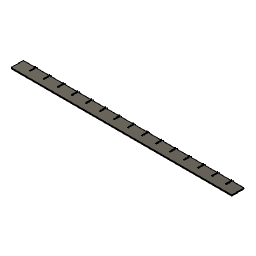
Matrix_Y (Autodesk Fusion 360 design; units mm, degrees)
Autodesk Fusion 360 part; units mm, degrees
other "Base Mesh Feature1"
sketch "Sketch1" plane through (0, 0, 0) normal (0, 0, 1) x (1, 0, 0)
  line L0 (0, 0) -> (252, 0)
  line L1 (252, 0) -> (252, 14)
  line L2 (0, 14) -> (0, 0)
  line L3 (14.5, 15) -> (14.5, 7.35)
  line L4 (14.5, 7.35) -> (13.5, 7.35)
  line L5 (13.5, 7.35) -> (13.5, 15)
  line L6 (13.5, 15) -> (12.5, 15)
  line L7 (30.5, 15) -> (30.5, 7.35)
  line L8 (30.5, 7.35) -> (29.5, 7.35)
  line L9 (29.5, 7.35) -> (29.5, 15)
  line L10 (46.5, 15) -> (46.5, 7.35)
  line L11 (46.5, 7.35) -> (45.35, 7.35)
  line L12 (45.35, 7.35) -> (45.35, 15)
  line L13 (62.5, 15) -> (62.5, 7.35)
  line L14 (62.5, 7.35) -> (61.35, 7.35)
  line L15 (61.35, 7.35) -> (61.35, 15)
  line L16 (78.5, 15) -> (78.5, 7.35)
  line L17 (78.5, 7.35) -> (77.35, 7.35)
  line L18 (77.35, 7.35) -> (77.35, 15)
  line L19 (94.5, 15) -> (94.5, 7.35)
  line L20 (94.5, 7.35) -> (93.35, 7.35)
  line L21 (93.35, 7.35) -> (93.35, 15)
  line L22 (110.5, 15) -> (110.5, 7.35)
  line L23 (110.5, 7.35) -> (109.35, 7.35)
  line L24 (109.35, 7.35) -> (109.35, 15)
  line L25 (126.5, 15) -> (126.5, 7.35)
  line L26 (126.5, 7.35) -> (125.35, 7.35)
  line L27 (125.35, 7.35) -> (125.35, 15)
  line L28 (142.5, 15) -> (142.5, 7.35)
  line L29 (142.5, 7.35) -> (141.35, 7.35)
  line L30 (141.35, 7.35) -> (141.35, 15)
  line L31 (158.5, 15) -> (158.5, 7.35)
  line L32 (158.5, 7.35) -> (157.35, 7.35)
  line L33 (157.35, 7.35) -> (157.35, 15)
  line L34 (174.5, 15) -> (174.5, 7.35)
  line L35 (174.5, 7.35) -> (173.35, 7.35)
  line L36 (173.35, 7.35) -> (173.35, 15)
  line L37 (190.5, 15) -> (190.5, 7.35)
  line L38 (190.5, 7.35) -> (189.35, 7.35)
  line L39 (189.35, 7.35) -> (189.35, 15)
  line L40 (206.5, 15) -> (206.5, 7.35)
  line L41 (206.5, 7.35) -> (205.35, 7.35)
  line L42 (205.35, 7.35) -> (205.35, 15)
  line L43 (222.5, 15) -> (222.5, 7.35)
  line L44 (222.5, 7.35) -> (221.35, 7.35)
  line L45 (221.35, 7.35) -> (221.35, 15)
  line L46 (238.5, 15) -> (238.5, 7.35)
  line L47 (238.5, 7.35) -> (237.35, 7.35)
  line L48 (237.35, 7.35) -> (237.35, 15)
  line L49 (239.5, 15) -> (238.5, 15)
  line L50 (223.5, 15) -> (223.5, 14)
  line L51 (223.5, 14) -> (236.35, 14)
  line L52 (236.35, 14) -> (236.35, 15)
  line L53 (252, 14) -> (239.5, 14)
  line L54 (239.5, 14) -> (239.5, 15)
  line L55 (220.35, 15) -> (220.35, 14)
  line L56 (220.35, 14) -> (207.5, 14)
  line L57 (207.5, 14) -> (207.5, 15)
  line L58 (237.35, 15) -> (236.35, 15)
  line L59 (223.5, 15) -> (222.5, 15)
  line L60 (221.35, 15) -> (220.35, 15)
  line L61 (207.5, 15) -> (206.5, 15)
  line L62 (204.35, 15) -> (204.35, 14)
  line L63 (204.35, 14) -> (191.5, 14)
  line L64 (191.5, 14) -> (191.5, 15)
  line L65 (205.35, 15) -> (204.35, 15)
  line L66 (191.5, 15) -> (190.5, 15)
  line L67 (188.35, 15) -> (188.35, 14)
  line L68 (188.35, 14) -> (175.5, 14)
  line L69 (175.5, 14) -> (175.5, 15)
  line L70 (189.35, 15) -> (188.35, 15)
  line L71 (175.5, 15) -> (174.5, 15)
  line L72 (172.35, 15) -> (172.35, 14)
  line L73 (172.35, 14) -> (159.5, 14)
  line L74 (159.5, 14) -> (159.5, 15)
  line L75 (173.35, 15) -> (172.35, 15)
  line L76 (159.5, 15) -> (158.5, 15)
  line L77 (156.35, 15) -> (156.35, 14)
  line L78 (156.35, 14) -> (143.5, 14)
  line L79 (143.5, 14) -> (143.5, 15)
  line L80 (157.35, 15) -> (156.35, 15)
  line L81 (143.5, 15) -> (142.5, 15)
  line L82 (140.35, 15) -> (140.35, 14)
  line L83 (140.35, 14) -> (127.5, 14)
  line L84 (127.5, 14) -> (127.5, 15)
  line L85 (141.35, 15) -> (140.35, 15)
  line L86 (127.5, 15) -> (126.5, 15)
  line L87 (124.35, 15) -> (124.35, 14)
  line L88 (124.35, 14) -> (111.5, 14)
  line L89 (111.5, 14) -> (111.5, 15)
  line L90 (125.35, 15) -> (124.35, 15)
  line L91 (111.5, 15) -> (110.5, 15)
  line L92 (108.35, 15) -> (108.35, 14)
  line L93 (108.35, 14) -> (95.5, 14)
  line L94 (95.5, 14) -> (95.5, 15)
  line L95 (109.35, 15) -> (108.35, 15)
  line L96 (95.5, 15) -> (94.5, 15)
  line L97 (92.35, 15) -> (92.35, 14)
  line L98 (92.35, 14) -> (79.5, 14)
  line L99 (79.5, 14) -> (79.5, 15)
  line L100 (93.35, 15) -> (92.35, 15)
  line L101 (79.5, 15) -> (78.5, 15)
  line L102 (76.35, 15) -> (76.35, 14)
  line L103 (76.35, 14) -> (63.5, 14)
  line L104 (63.5, 14) -> (63.5, 15)
  line L105 (77.35, 15) -> (76.35, 15)
  line L106 (63.5, 15) -> (62.5, 15)
  line L107 (60.35, 15) -> (60.35, 14)
  line L108 (60.35, 14) -> (47.5, 14)
  line L109 (47.5, 14) -> (47.5, 15)
  line L110 (61.35, 15) -> (60.35, 15)
  line L111 (47.5, 15) -> (46.5, 15)
  line L112 (44.35, 15) -> (44.35, 14)
  line L113 (44.35, 14) -> (31.5, 14)
  line L114 (31.5, 14) -> (31.5, 15)
  line L115 (45.35, 15) -> (44.35, 15)
  line L116 (31.5, 15) -> (30.5, 15)
  line L117 (28.5, 15) -> (28.5, 14)
  line L118 (28.5, 14) -> (15.5, 14)
  line L119 (15.5, 14) -> (15.5, 15)
  line L120 (29.5, 15) -> (28.5, 15)
  line L121 (15.5, 15) -> (14.5, 15)
  line L122 (0, 14) -> (12.5, 14)
  line L123 (12.5, 14) -> (12.5, 15)
  dimension "d2" = 252
  dimension "d5" = 1
  dimension "d6" = 15
  dimension "d7" = 1
  dimension "d8" = 14.85
  dimension "d9" = 1.15
  dimension "d10" = 14.85
  dimension "d11" = 1.15
  dimension "d12" = 14.85
  dimension "d13" = 1.15
  dimension "d14" = 14.85
  dimension "d15" = 1.15
  dimension "d16" = 14.85
  dimension "d17" = 1.15
  dimension "d18" = 14.85
  dimension "d19" = 1.15
  dimension "d20" = 14.85
  dimension "d21" = 1.15
  dimension "d22" = 14.85
  dimension "d23" = 1.15
  dimension "d24" = 14.85
  dimension "d25" = 1.15
  dimension "d26" = 14.85
  dimension "d27" = 1.15
  dimension "d28" = 14.85
  dimension "d29" = 1.15
  dimension "d30" = 14.85
  dimension "d31" = 1.15
  dimension "d32" = 14.85
  dimension "d33" = 1.15
  dimension "d36" = 7.65
  dimension "d37" = 7.65
  dimension "d38" = 7.65
  dimension "d39" = 7.65
  dimension "d40" = 7.65
  dimension "d41" = 7.65
  dimension "d42" = 7.65
  dimension "d43" = 7.65
  dimension "d44" = 7.65
  dimension "d45" = 7.65
  dimension "d46" = 7.65
  dimension "d47" = 7.65
  dimension "d48" = 7.65
  dimension "d49" = 7.65
  dimension "d50" = 7.65
  dimension "d51" = 1
  dimension "d52" = 1
  dimension "d53" = 1
  dimension "d54" = 1
  dimension "d55" = 1
  dimension "d56" = 1
  dimension "d57" = 1
  dimension "d58" = 1
  dimension "d59" = 1
  dimension "d60" = 1
  dimension "d61" = 1
  dimension "d62" = 1
  dimension "d63" = 1
  dimension "d64" = 1
  dimension "d65" = 1
  dimension "d66" = 1
  dimension "d67" = 1
  dimension "d68" = 1
  dimension "d69" = 1
  dimension "d70" = 1
  dimension "d71" = 1
  dimension "d72" = 1
  dimension "d73" = 1
  dimension "d74" = 1
  dimension "d75" = 1
  dimension "d76" = 1
  dimension "d77" = 1
  dimension "d78" = 1
  dimension "d79" = 1
  dimension "d80" = 1
  dimension "d81" = 1
  dimension "d82" = 1
  dimension "d83" = 1
  dimension "d84" = 1
  dimension "d85" = 1
  dimension "d86" = 1
  dimension "d87" = 1
  dimension "d88" = 1
  dimension "d89" = 1
  dimension "d90" = 1
  dimension "d91" = 1
  dimension "d92" = 1
  dimension "d93" = 1
  dimension "d94" = 1
  dimension "d95" = 12.5
  dimension "d96" = 12.5
  constraint horizontal L0
  constraint vertical L1
  constraint horizontal L49
  constraint vertical L2
  constraint coincident L0.start L2.end
  constraint vertical L3
  constraint horizontal L4
  constraint vertical L5
  constraint coincident L5.end L49
  constraint collinear L6 L49
  constraint vertical L7
  constraint horizontal L8
  constraint vertical L9
  constraint coincident L9.end L49
  constraint vertical L10
  constraint horizontal L11
  constraint vertical L12
  constraint coincident L12.end L49
  constraint vertical L13
  constraint horizontal L14
  constraint vertical L15
  constraint coincident L15.end L49
  constraint vertical L16
  constraint horizontal L17
  constraint vertical L18
  constraint coincident L18.end L49
  constraint vertical L19
  constraint horizontal L20
  constraint vertical L21
  constraint coincident L21.end L49
  constraint vertical L22
  constraint horizontal L23
  constraint vertical L24
  constraint coincident L24.end L49
  constraint vertical L25
  constraint horizontal L26
  constraint vertical L27
  constraint coincident L27.end L49
  constraint vertical L28
  constraint horizontal L29
  constraint vertical L30
  constraint coincident L30.end L49
  constraint vertical L31
  constraint horizontal L32
  constraint vertical L33
  constraint coincident L33.end L49
  constraint vertical L34
  constraint horizontal L35
  constraint vertical L36
  constraint coincident L36.end L49
  constraint vertical L37
  constraint horizontal L38
  constraint vertical L39
  constraint coincident L39.end L49
  constraint vertical L40
  constraint horizontal L41
  constraint vertical L42
  constraint coincident L42.end L49
  constraint vertical L43
  constraint horizontal L44
  constraint vertical L45
  constraint coincident L45.end L49
  constraint vertical L46
  constraint horizontal L47
  constraint vertical L48
  constraint coincident L48.end L49
  constraint collinear L49 L120
  constraint collinear L49 L115
  constraint collinear L49 L110
  constraint collinear L49 L105
  constraint collinear L49 L100
  constraint collinear L49 L95
  constraint collinear L49 L90
  constraint collinear L49 L85
  constraint collinear L49 L80
  constraint collinear L49 L75
  constraint collinear L49 L70
  constraint collinear L49 L65
  constraint collinear L49 L60
  constraint collinear L49 L58
  constraint vertical L50
  constraint horizontal L51
  constraint vertical L52
  constraint horizontal L53
  constraint vertical L54
  constraint vertical L55
  constraint horizontal L56
  constraint vertical L57
  constraint coincident L57.end L60
  constraint collinear L58 L59
  constraint collinear L60 L61
  constraint vertical L62
  constraint horizontal L63
  constraint vertical L64
  constraint coincident L64.end L65
  constraint collinear L65 L66
  constraint vertical L67
  constraint horizontal L68
  constraint vertical L69
  constraint coincident L69.end L70
  constraint collinear L70 L71
  constraint vertical L72
  constraint horizontal L73
  constraint vertical L74
  constraint coincident L74.end L75
  constraint collinear L75 L76
  constraint vertical L77
  constraint horizontal L78
  constraint vertical L79
  constraint coincident L79.end L80
  constraint collinear L80 L81
  constraint vertical L82
  constraint horizontal L83
  constraint vertical L84
  constraint coincident L84.end L85
  constraint collinear L85 L86
  constraint vertical L87
  constraint horizontal L88
  constraint vertical L89
  constraint coincident L89.end L90
  constraint collinear L90 L91
  constraint vertical L92
  constraint horizontal L93
  constraint vertical L94
  constraint coincident L94.end L95
  constraint collinear L95 L96
  constraint vertical L97
  constraint horizontal L98
  constraint vertical L99
  constraint coincident L99.end L100
  constraint collinear L100 L101
  constraint vertical L102
  constraint horizontal L103
  constraint vertical L104
  constraint coincident L104.end L105
  constraint collinear L105 L106
  constraint vertical L107
  constraint horizontal L108
  constraint vertical L109
  constraint coincident L109.end L110
  constraint collinear L110 L111
  constraint vertical L112
  constraint horizontal L113
  constraint vertical L114
  constraint coincident L114.end L115
  constraint collinear L115 L116
  constraint vertical L117
  constraint horizontal L118
  constraint vertical L119
  constraint coincident L119.end L120
  constraint collinear L120 L121
  constraint horizontal L122
  constraint vertical L123
  measures "d2" distance of L0.start L0.end
  measures "d5" distance of L5.end L3.start
  measures "d6" distance of L3.start L9.end
  measures "d7" distance of L9.end L7.start
  measures "d8" distance of L7.start L12.end
  measures "d9" distance of L12.end L10.start
  measures "d10" distance of L10.start L15.end
  measures "d11" distance of L15.end L13.start
  measures "d12" distance of L13.start L18.end
  measures "d13" distance of L18.end L16.start
  measures "d14" distance of L16.start L21.end
  measures "d15" distance of L21.end L19.start
  measures "d16" distance of L19.start L24.end
  measures "d17" distance of L24.end L22.start
  measures "d18" distance of L22.start L27.end
  measures "d19" distance of L27.end L25.start
  measures "d20" distance of L25.start L30.end
  measures "d21" distance of L30.end L28.start
  measures "d22" distance of L28.start L33.end
  measures "d23" distance of L33.end L31.start
  measures "d24" distance of L31.start L36.end
  measures "d25" distance of L36.end L34.start
  measures "d26" distance of L34.start L39.end
  measures "d27" distance of L39.end L37.start
  measures "d28" distance of L37.start L42.end
  measures "d29" distance of L42.end L40.start
  measures "d30" distance of L40.start L45.end
  measures "d31" distance of L45.end L43.start
  measures "d32" distance of L43.start L48.end
  measures "d33" distance of L48.end L46.start
  measures "d36" distance of L5.end L4.end
  measures "d37" distance of L9.end L8.end
  measures "d38" distance of L12.end L11.end
  measures "d39" distance of L15.end L14.end
  measures "d40" distance of L18.end L17.end
  measures "d41" distance of L21.end L20.end
  measures "d42" distance of L24.end L23.end
  measures "d43" distance of L27.end L26.end
  measures "d44" distance of L30.end L29.end
  measures "d45" distance of L33.end L32.end
  measures "d46" distance of L36.end L35.end
  measures "d47" distance of L39.end L38.end
  measures "d48" distance of L42.end L41.end
  measures "d49" distance of L45.end L44.end
  measures "d50" distance of L48.end L47.end
  measures "d51" distance of L43.start L50.start
  measures "d52" distance of L48.end L52.end
  measures "d53" distance of L52.end L51.end
  measures "d54" distance of L49.start L53.end
  measures "d55" distance of L46.start L49.start
  measures "d56" distance of L55.start L55.end
  measures "d57" distance of L40.start L57.end
  measures "d58" distance of L45.end L55.start
  measures "d59" distance of L64.end L63.end
  measures "d60" distance of L37.start L64.end
  measures "d61" distance of L42.end L62.start
  measures "d62" distance of L69.end L68.end
  measures "d63" distance of L34.start L69.end
  measures "d64" distance of L39.end L67.start
  measures "d65" distance of L74.end L73.end
  measures "d66" distance of L36.end L72.start
  measures "d67" distance of L31.start L74.end
  measures "d68" distance of L28.start L79.end
  measures "d69" distance of L33.end L77.start
  measures "d70" distance of L84.end L83.end
  measures "d71" distance of L30.end L82.start
  measures "d72" distance of L25.start L84.end
  measures "d73" distance of L89.end L88.end
  measures "d74" distance of L22.start L89.end
  measures "d75" distance of L27.end L87.start
  measures "d76" distance of L94.end L93.end
  measures "d77" distance of L24.end L92.start
  measures "d78" distance of L19.start L94.end
  measures "d79" distance of L99.end L98.end
  measures "d80" distance of L21.end L97.start
  measures "d81" distance of L16.start L99.end
  measures "d82" distance of L104.end L103.end
  measures "d83" distance of L18.end L102.start
  measures "d84" distance of L13.start L104.end
  measures "d85" distance of L109.end L108.end
  measures "d86" distance of L15.end L107.start
  measures "d87" distance of L10.start L109.end
  measures "d88" distance of L114.end L113.end
  measures "d89" distance of L7.start L114.end
  measures "d90" distance of L12.end L112.start
  measures "d91" distance of L119.end L118.end
  measures "d92" distance of L9.end L117.start
  measures "d93" distance of L3.start L119.end
  measures "d94" distance of L5.end L6.end
  measures "d95" distance of L2.start L122.end
  measures "d96" distance of L1.end L53.end
other "Modify1"
other "Modify2"
other "Modify3"
extrude "Extrude1" add sketch "Sketch1" along normal blind 1
